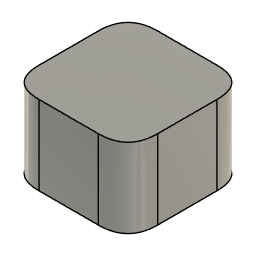
squircle_v2 (Autodesk Fusion 360 design; units mm, degrees)
Autodesk Fusion 360 part; units mm, degrees
sketch "profile" plane through (0, 0, 0) normal (0, 0, 1) x (1, 0, 0)
  line L0 (15, -15) -> (-15, -15)
  line L1 (-15, -15) -> (-15, 15)
  line L2 (-15, 15) -> (15, 15)
  line L3 (15, 15) -> (15, -15)
  line L4 (15, -15) -> (-15, 15) construction
  line L5 (-15, -15) -> (15, 15) construction
  spline S0 degree 2 poles (-15, 7.5) (-15, 15) (-7.5, 15) knots 0 0 0 1.185854 1.185854 1.185854
  line L6 (-15, 0) -> (-15, 7.5)
  line L7 (-7.5, 15) -> (0, 15)
  line L8 (0, 15) -> (0, 0)
  line L9 (-15, 0) -> (0, 0)
  dimension "d1" = 30
  dimension "d4" = 7.5
  constraint horizontal L0
  constraint perpendicular L0 L1
  constraint parallel L0 L2
  constraint parallel L1 L3
  constraint coincident L4 L8.end
  constraint coincident L5 L8.end
  constraint coincident L8.end L9.end
  constraint equal L1 L2
  constraint coincident L1.end L2.start
  constraint midpoint L1 L6.start
  constraint parallel L1 L6
  constraint midpoint L2 L7.end
  constraint equal L6 L7
  measures "d1" distance of L1.end L2.end
  measures "d4" distance of S0.start L6.start
extrude "Extrude1" add sketch "profile" along normal blind 20 contours L1 L2 S0 L6 L7 L8 L9
mirror "Mirror1" about plane through (0, 0, 0) normal (1, 0, 0) of bodies 1 merged
mirror "Mirror2" about plane through (0, 0, 0) normal (0, 1, 0) of bodies 1 merged
equation "d4 = d1 / 4"
named bodies: "squircle"
